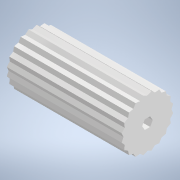
# Autodesk Inventor part: SolidRollerNoPulley
Saved by Autodesk Inventor 2021 (Build 250183000, 183)
## iProperties
Created: 2021-05-21
Part Number: SolidRollerNoPulley
Material: PC/ABS Plastic
Document SubType Name: Modeling
Designer: sami8
Density: 0.357273 g/cm^3
Appearance: Smooth - White
Author: sami8
Autodesk Inventor part; units mm, degrees
ref_plane "YZ Plane" through (0, 0, 0) normal (1, 0, 0) x (0, 1, 0)
ref_plane "XZ Plane" through (0, 0, 0) normal (0, 1, 0) x (-1, 0, 0)
ref_plane "XY Plane" through (0, 0, 0) normal (0, 0, 1) x (1, 0, 0)
sketch "Sketch1" plane through (0, 0, 0) normal (1, 0, 0) x (0, 1, 0)
  circle A0 centre (0, 0) radius 14.75 construction
  line L0 (2.6, -1.5011) -> (0, -3.0022)
  line L1 (0, -3.0022) -> (-2.6, -1.5011)
  line L2 (-2.6, -1.5011) -> (-2.6, 1.5011)
  line L3 (-2.6, 1.5011) -> (0, 3.0022)
  line L4 (0, 3.0022) -> (2.6, 1.5011)
  line L5 (2.6, 1.5011) -> (2.6, -1.5011)
  line L6 (14.5684, 2.3074) -> (14.5684, -2.3074) construction
  line L7 (14.5684, 2.3074) -> (0, 0) construction
  line L8 (0, 0) -> (14.5684, -2.3074) construction
  line L9 (14.5684, 2.3074) -> (13.5684, 0)
  line L10 (13.5684, 0) -> (14.5684, -2.3074)
  line L11 (13.5684, 0) -> (14.5684, 0) construction
  line L12 (13.1423, 6.6964) -> (12.9043, 4.1929)
  line L13 (12.9043, 4.1929) -> (14.5684, 2.3074)
  line L14 (10.4298, 10.4298) -> (10.9771, 7.9753)
  line L15 (10.9771, 7.9753) -> (13.1423, 6.6964)
  line L16 (6.6964, 13.1423) -> (7.9753, 10.9771)
  line L17 (7.9753, 10.9771) -> (10.4298, 10.4298)
  line L18 (2.3074, 14.5684) -> (4.1929, 12.9043)
  line L19 (4.1929, 12.9043) -> (6.6964, 13.1423)
  line L20 (-2.3074, 14.5684) -> (0, 13.5684)
  line L21 (0, 13.5684) -> (2.3074, 14.5684)
  line L22 (-6.6964, 13.1423) -> (-4.1929, 12.9043)
  line L23 (-4.1929, 12.9043) -> (-2.3074, 14.5684)
  line L24 (-10.4298, 10.4298) -> (-7.9753, 10.9771)
  line L25 (-7.9753, 10.9771) -> (-6.6964, 13.1423)
  line L26 (-13.1423, 6.6964) -> (-10.9771, 7.9753)
  line L27 (-10.9771, 7.9753) -> (-10.4298, 10.4298)
  line L28 (-14.5684, 2.3074) -> (-12.9043, 4.1929)
  line L29 (-12.9043, 4.1929) -> (-13.1423, 6.6964)
  line L30 (-14.5684, -2.3074) -> (-13.5684, 0)
  line L31 (-13.5684, 0) -> (-14.5684, 2.3074)
  line L32 (-13.1423, -6.6964) -> (-12.9043, -4.1929)
  line L33 (-12.9043, -4.1929) -> (-14.5684, -2.3074)
  line L34 (-10.4298, -10.4298) -> (-10.9771, -7.9753)
  line L35 (-10.9771, -7.9753) -> (-13.1423, -6.6964)
  line L36 (-6.6964, -13.1423) -> (-7.9753, -10.9771)
  line L37 (-7.9753, -10.9771) -> (-10.4298, -10.4298)
  line L38 (-2.3074, -14.5684) -> (-4.1929, -12.9043)
  line L39 (-4.1929, -12.9043) -> (-6.6964, -13.1423)
  line L40 (2.3074, -14.5684) -> (0, -13.5684)
  line L41 (0, -13.5684) -> (-2.3074, -14.5684)
  line L42 (6.6964, -13.1423) -> (4.1929, -12.9043)
  line L43 (4.1929, -12.9043) -> (2.3074, -14.5684)
  line L44 (10.4298, -10.4298) -> (7.9753, -10.9771)
  line L45 (7.9753, -10.9771) -> (6.6964, -13.1423)
  line L46 (13.1423, -6.6964) -> (10.9771, -7.9753)
  line L47 (10.9771, -7.9753) -> (10.4298, -10.4298)
  line L48 (14.5684, -2.3074) -> (12.9043, -4.1929)
  line L49 (12.9043, -4.1929) -> (13.1423, -6.6964)
  dimension "d0" = 29.5
  dimension "d1" = 5.2
  dimension "d2" = 18
  dimension "d3" = 1
  dimension "d6" = 360
  constraints: 100 end point, 2 coincident, 2 point on circle, 2 vertical, 1 centre point, 1 horizontal, 1 midpoint, 114 other
  measures "d0" diameter of A0
  measures "d1" distance between parallel lines of L5 L2
  measures "d2" angle of L8 L7
  measures "d3" distance of L9.end L11.end
extrude "Extrusion1" add sketch "Sketch1" along normal mid plane 60
body "Solid1"
